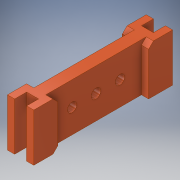
# Autodesk Inventor part: МД.001.1003 - Каретка
Saved by Autodesk Inventor 2019 (Build 230136000, 136)
## iProperties
Created: 2020-01-02
Part Number: МД.001.1003 - Каретка
Material: Пластик АБС
Document SubType Name: Modeling
Designer: Петров Иван
Density: 1.06 g/cm^3
Appearance: Гладкий — светло-оранжевый
Author: Петров Иван
Autodesk Inventor part; units mm, degrees
ref_plane "YZ Plane" through (0, 0, 0) normal (1, 0, 0) x (0, 1, 0)
ref_plane "XZ Plane" through (0, 0, 0) normal (0, 1, 0) x (-1, 0, 0)
ref_plane "XY Plane" through (0, 0, 0) normal (0, 0, 1) x (1, 0, 0)
sketch "Эскиз1" plane through (0, 0, 0) normal (0, 1, 0) x (-1, 0, 0)
  line L0 (-2.5, 24) -> (2.5, 24)
  line L1 (2.5, 24) -> (2.5, -24)
  line L2 (2.5, -24) -> (-2.5, -24)
  line L3 (-2.5, -24) -> (-2.5, 24)
  line L4 (-2.5, 29) -> (2.5, 29)
  line L5 (2.5, 29) -> (2.5, -29)
  line L6 (2.5, -29) -> (-2.5, -29)
  line L7 (-2.5, -29) -> (-2.5, 29)
  line L8 (2.5, 29) -> (5.5, 29)
  line L9 (5.5, 29) -> (5.5, 19)
  line L10 (5.5, 19) -> (2.5, 19)
  line L11 (2.5, 19) -> (2.5, 29)
  line L12 (-2.5, 19) -> (-5.5, 19)
  line L13 (-5.5, 19) -> (-5.5, 29)
  line L14 (-5.5, 29) -> (-2.5, 29)
  line L15 (-2.5, 29) -> (-2.5, 19)
  line L16 (2.5, -29) -> (5.5, -29)
  line L17 (5.5, -29) -> (5.5, -19)
  line L18 (5.5, -19) -> (2.5, -19)
  line L19 (2.5, -19) -> (2.5, -29)
  line L20 (-2.5, -29) -> (-5.5, -29)
  line L21 (-5.5, -29) -> (-5.5, -19)
  line L22 (-5.5, -19) -> (-2.5, -19)
  line L23 (-2.5, -19) -> (-2.5, -29)
  point P0 (0, 0)
  dimension "d3" = 3
  dimension "d4" = 10
  dimension "d5" = 3
  dimension "d6" = 10
  dimension "d7" = 3
  dimension "d8" = 10
  dimension "d9" = 3
  dimension "d10" = 10
  constraints: 48 end point, 12 parallel, 6 horizontal, 6 perpendicular, 2 point on line
  measures "d3" distance of L9.end L10.end
  measures "d4" distance of L8.end L9.end
  measures "d5" distance of L13.end L14.end
  measures "d6" distance of L12.end L13.end
  measures "d7" distance of L18.end L17.end
  measures "d8" distance of L17.end L16.end
  measures "d9" distance of L21.end L22.end
  measures "d10" distance of L20.end L21.end
extrude "Выдавливание1" add sketch "Эскиз1" along normal blind 20 contours L0 L1 L2 L3 | L3 L12 L13 L14 L7 | L5 L8 L9 L10 L1 | L3 L7 L20 L21 L22 | L18 L17 L16 L5 L1
sketch "Эскиз2" plane through (2.5, 0, 19) normal (1, 0, 0) x (0, 0, -1)
  line L0 (19, 0) -> (19, 20)
  line L1 (0, 20) -> (38, 20) projected
  circle A0 centre (19, 10) radius 2
  dimension "d13" = 4
  constraints: 2 end point, 2 midpoint, 1 centre point
  measures "d13" diameter of A0
extrude "Выдавливание2" cut sketch "Эскиз2" against normal blind 35
chamfer "Фаска1" distance 2 angle 45 7 edges at (-4, 20, -19) (-4, 0, -19) (4, 20, -19) (4, 20, 19) (-4, 20, 19) (-4, 0, 19) (4, 0, 19)
sketch "Эскиз3" plane through (2.5, 0, -19) normal (1, 0, 0) x (0, 0, -1)
  circle A0 centre (-19, 10) radius 2 projected
  line L0 (-19, 10) -> (-9, 10)
  line L1 (-19, 10) -> (-29, 10)
  circle A1 centre (-29, 10) radius 1.95
  circle A2 centre (-9, 10) radius 1.95
  point P0 (-19, 0)
  dimension "d19" = 10
  dimension "d20" = 10
  dimension "d21" = 3.9
  dimension "d22" = 3.9
  constraints: 4 end point, 2 centre point, 2 coincident, 2 horizontal
  measures "d19" distance of L0.start L0.end
  measures "d20" distance of L0.start L1.end
  measures "d21" diameter of A1
  measures "d22" diameter of A2
extrude "Выдавливание3" cut sketch "Эскиз3" against normal blind 22 contours A1 | A2
